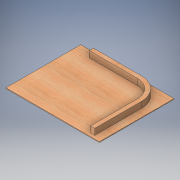
# Autodesk Inventor part: ShooterBase
Saved by Autodesk Inventor 2016 (Build 200138000, 138)
## iProperties
Created: 2015-07-21
Part Number: ShooterBase
Material: Wood (Birch)
Document SubType Name: Modeling
Designer: steele
Density: 0.55 g/cm^3
Appearance: Birch - Natural Polished
Author: steele
Autodesk Inventor part; units mm, degrees
ref_plane "YZ Plane" through (0, 0, 0) normal (1, 0, 0) x (0, 1, 0)
ref_plane "XZ Plane" through (0, 0, 0) normal (0, 1, 0) x (-1, 0, 0)
ref_plane "XY Plane" through (0, 0, 0) normal (0, 0, 1) x (1, 0, 0)
sketch "Sketch1" plane through (0, 0, 0) normal (0, 1, 0) x (-1, 0, 0)
  line L0 (-381, 304.8) -> (-381, -304.8)
  line L1 (-381, -304.8) -> (381, -304.8)
  line L2 (381, -304.8) -> (381, 304.8)
  line L3 (381, 304.8) -> (-381, 304.8)
  line L4 (-381, 304.8) -> (381, -304.8) construction
  line L5 (-381, -304.8) -> (381, 304.8) construction
  point P0 (0, 0)
  dimension "width" = 609.6
  dimension "length" = 762
  constraints: 12 end point, 2 midpoint, 2 parallel, 1 perpendicular, 1 vertical
  measures "width" distance of L0.start L0.end
  measures "length" distance of L2.end L0.start
extrude "Extrusion1" add sketch "Sketch1" against normal blind 6.35
ref_plane "Work Plane1" through (-381, 0, 274.6375) normal (0, 0, 1) x (1, 0, 0)
sketch "Sketch2" plane through (0, 0, 0) normal (0, 1, 0) x (1, 0, 0)
  line L0 (-254.5026, 247.65) -> (138.8237, 247.65)
  line L1 (284.8737, 101.6) -> (284.8737, -279.4)
  arc A0 (284.8737, 101.6) -> (138.8237, 247.65) centre (138.8237, 101.6) ccw
  line L2 (-381, -304.8) -> (381, -304.8) projected
  point P0 (0, 0)
  dimension "d4" = 292.1
  dimension "d5" = 381
  dimension "d6" = 558.8
  dimension "d10" = 25.4
  constraints: 4 end point, 2 point on circle, 2 tangent, 1 centre point, 1 horizontal, 1 perpendicular
  measures "d4" diameter of A0
  measures "d5" distance of L1.start L1.end
  measures "d6" distance of L0.start L1.start
  measures "d10" distance from line of L1.end L2
sketch "Sketch3" plane through (-381, 0, 274.6375) normal (0, 0, 1) x (1, 0, 0)
  line L0 (665.6905, 0) -> (699.5621, 0)
  line L1 (699.5621, 0) -> (699.5621, 50.8385)
  line L2 (699.5621, 50.8385) -> (665.6905, 50.8385)
  line L3 (665.6905, 50.8385) -> (665.6905, 0)
  point P0 (381, 0)
  constraints: 8 end point, 2 parallel, 1 horizontal, 1 perpendicular
sweep "Sweep1" add profiles "Sketch3" path "Sketch2" path curves L1 A0 L0
body "Solid1"
